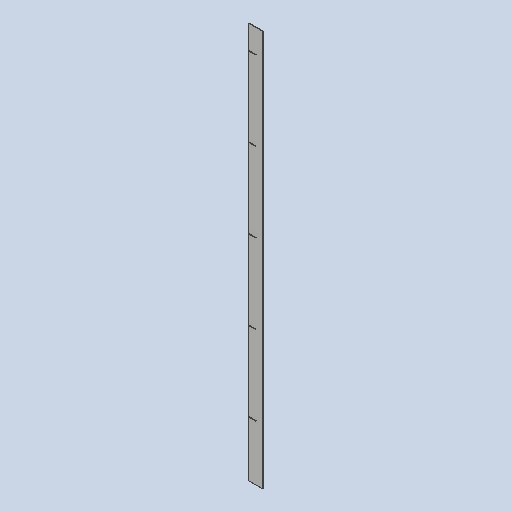
# Autodesk Inventor part: BSH 041 stringer 1
Saved by Autodesk Inventor 2025 (Build 290162010, 162A)
## iProperties
Created: 2024-07-23
Part Number: BSH 041 stringer 1
Material: 09g2s
Document SubType Name: Sheet Metal
Designer: admin
Density: 7.85 g/cm^3
Sheet Metal Rule: AISI304 3mm Die 32
Sheet Metal Width: 0,000 mm
Sheet Metal Length: 0,000 mm
Sheet Metal Area: 0,000 mm^2
Appearance: Default
Author: admin
Autodesk Inventor part; units mm, degrees
ref_plane "YZ Plane" through (0, 0, 0) normal (1, 0, 0) x (0, 1, 0)
ref_plane "XZ Plane" through (0, 0, 0) normal (0, 1, 0) x (-1, 0, 0)
ref_plane "XY Plane" through (0, 0, 0) normal (0, 0, 1) x (1, 0, 0)
sketch "Sketch6" plane through (0, 0, 0) normal (0, 1, 0) x (-1, 0, 0)
  line L0 (0, 0) -> (-90.8346, 0)
  line L1 (-90.8346, 0) -> (-90.8346, 2500)
  line L2 (-90.8346, 2500) -> (0, 2500)
  line L3 (0, 2500) -> (0, 0)
  dimension "d26" = 90.8346
  dimension "d27" = 2500
  measures "d26" distance of L1.end L2.end
  measures "d27" distance of L0.end L1.end
extrude "Plate4" add sketch "Sketch6" along normal blind 3
sketch "Sketch7" plane through (0, 0, 0) normal (0, -1, 0) x (1, 0, 0)
  line L0 (0, 2500) -> (90.8346, 2500) projected
  line L1 (0, 0) -> (0, 2500) projected
  line L2 (90.8346, 0) -> (0, 0) projected
  line L3 (90.8346, 2500) -> (90.8346, 0) projected
  line L4 (0, 351.6) -> (46.4173, 351.6)
  line L5 (46.4173, 351.6) -> (46.4173, 348.4)
  line L6 (46.4173, 348.4) -> (0, 348.4)
  line L7 (0, 348.4) -> (0, 351.6)
  point P0 (0, 348.4)
  point P1 (0, 200)
  point P2 (46.4173, 200)
  point P3 (0, 348.4)
  dimension "d29" = 46.4173
  dimension "d30" = 3.2
  dimension "d31" = 348.4
  constraints: 8 end point, 2 parallel, 1 horizontal, 1 perpendicular, 1 point on line
  measures "d29" distance of L5.end L6.end
  measures "d30" distance of L4.end L5.end
  measures "d31" distance between parallel lines of L2 L6
extrude "Extrusion2" cut sketch "Sketch7" against normal through all contours L4 L5 L6 L1
pattern_linear "Rectangular Pattern1" count 5 spacing 500 along (0, 0, 1) of "Extrusion2"
equation "\"d26\" = Stringer1_deep"
equation "\"d28\" = Thickness"
equation "\"BendReliefWidth\" = Thickness"
equation "\"BendReliefDepth\" = 0.5 * Thickness"
equation "\"CornerReliefSize\" = 4 * Thickness"
equation "\"MinimumRemnant\" = 2 * Thickness"
equation "\"TransitionRadius\" = BendRadius"
equation "\"JacobiRadiusSize\" = BendRadius"
equation "\"GapSize\" = Thickness"
equation "\"Stringer1_deep\" = 90.834574"
equation "\"Thickness\" = 3"
equation "\"BendRadius\" = 5"
body "Solid2"
